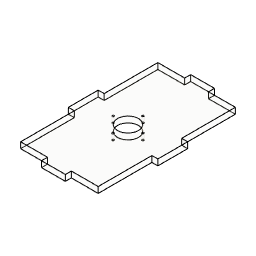
bottom_plate (Autodesk Fusion 360 design; units mm, degrees)
Autodesk Fusion 360 part; units mm, degrees
note: some values were not read from the file. Set by a fixed rule: which sketch regions a step uses.
sketch "Esquisse1" plane through (0, 0, 0) normal (0, 0, 1) x (1, 0, 0)
  line L0 (75, -125) -> (-75, -125) construction
  line L1 (-75, -125) -> (-75, 125) construction
  line L2 (-75, 125) -> (75, 125) construction
  line L3 (75, 125) -> (75, -125) construction
  line L4 (75, -125) -> (-75, 125) construction
  line L5 (-75, -125) -> (75, 125) construction
  circle A0 centre (0, 0) radius 17.5
  circle A1 centre (0, 0) radius 25 construction
  circle A2 centre (0, 25) radius 1.6
  circle A3 centre (-25, 0) radius 1.6
  circle A4 centre (0, -25) radius 1.6
  circle A5 centre (25, 0) radius 1.6
  line L6 (0, 125) -> (0, -125)
  line L7 (-75, 0) -> (75, 0)
  line L8 (75, 125) -> (-75, 125) construction
  line L9 (-75, -125) -> (75, -125) construction
  line L10 (75, -125) -> (-75, -125) construction
  line L11 (-65, 115) -> (-65, 25)
  line L12 (-65, 25) -> (-75, 25)
  line L13 (-75, 25) -> (-75, -25)
  line L14 (-75, -25) -> (-65, -25)
  line L15 (-65, -25) -> (-65, -115)
  line L16 (65, 115) -> (65, 25)
  line L17 (65, 25) -> (75, 25)
  line L18 (75, -125) -> (75, 125) construction
  line L19 (75, -25) -> (65, -25)
  line L20 (65, -25) -> (65, -115)
  line L21 (75, 25) -> (75, -25)
  line L22 (-65, 115) -> (-20, 115)
  line L23 (-20, 115) -> (-20, 125)
  line L24 (20, 125) -> (-20, 125)
  line L25 (20, 125) -> (20, 115)
  line L26 (20, 115) -> (65, 115)
  line L27 (20, -125) -> (20, -115)
  line L28 (20, -115) -> (65, -115)
  line L29 (20, -125) -> (-20, -125)
  line L30 (-20, -115) -> (-20, -125)
  line L31 (-65, -115) -> (-20, -115)
  circle A6 centre (0, 0) radius 33.25 construction
  dimension "d1" = 150
  dimension "d2" = 250
  dimension "d3" = 35
  dimension "d5" = 3.2
  dimension "d9" = 50
  dimension "d14" = 40
  dimension "d15" = 10
  dimension "d16" = 10
  dimension "d17" = 66.5
  dimension "d18" = 50
  dimension "d25" = 10
  constraint horizontal L0
  constraint perpendicular L0 L1
  constraint parallel L0 L2
  constraint parallel L1 L3
  constraint coincident L4 A0.centre
  constraint coincident L5 A0.centre
  constraint coincident A0.centre A1.centre
  constraint coincident A1 A2.centre
  constraint coincident A1 A4.centre
  constraint coincident A1 A5.centre
  constraint equal A2 A5
  constraint equal A4 A5
  constraint equal A3 A4
  constraint midpoint L2 L6.start
  constraint midpoint L0 L6.end
  constraint midpoint L1 L7.start
  constraint midpoint L3 L7.end
  constraint coincident A2.centre L6
  constraint coincident A5.centre L7
  constraint coincident A4.centre L6
  constraint coincident A3.centre L7
  constraint coincident A1 A3.centre
  constraint symmetric L1.end L6 L2.end
  constraint symmetric L2.end L6 L1.end
  constraint symmetric L1.end L7 L0.end
  constraint symmetric L2.end L7 L0.start
  constraint symmetric L7 L2.end L0.start
  constraint symmetric L7 L1.end L0.end
  constraint perpendicular L8 L11
  constraint coincident L1 L12.end
  constraint perpendicular L1 L12
  constraint coincident L1 L13.end
  constraint perpendicular L13 L14
  constraint equal L12 L14
  constraint vertical L15
  constraint symmetric L7 L11.end L14.end
  constraint symmetric L0.end L6 L0.start
  constraint symmetric L6 L11.end L16.end
  constraint symmetric L6 L12.end L17.end
  constraint symmetric L6 L13.end L19.start
  constraint symmetric L6 L14.end L19.end
  constraint perpendicular L11 L22
  constraint coincident L8 L23.end
  constraint perpendicular L8 L23
  constraint coincident L2 L24.start
  constraint perpendicular L23 L24
  constraint perpendicular L24 L25
  constraint perpendicular L16 L26
  constraint symmetric L6 L23.end L24.start
  constraint equal L23 L25
  constraint vertical L16
  constraint symmetric L7 L11.start L15.end
  constraint symmetric L7 L22.end L30.start
  constraint symmetric L7 L23.end L29.end
  constraint symmetric L7 L24.start L27.start
  constraint symmetric L7 L25.end L27.end
  constraint symmetric L7 L16.start L20.end
  measures "d1" distance of L1.end L2.end
  measures "d2" distance of L0.end L1.end
  measures "d3" diameter of A0
  measures "d5" diameter of A2
  measures "d9" distance of L12 L14
  measures "d14" distance of L23 L25
  measures "d15" distance of L8 L22
  measures "d16" distance of L1 L11
  measures "d17" diameter of A6
  measures "d18" diameter of A1
extrude "Extrusion1" add sketch "Esquisse1" along normal blind 10 contours A0 A4 A5 L6 L7 L19 L20 L21 L27 L28 L29 | A0 A2 A5 L6 L7 L16 L17 L21 L24 L25 L26 | A0 A2 A3 L6 L7 L11 L12 L13 L22 L23 L24 | A0 A3 A4 L6 L7 L13 L14 L15 L29 L30 L31
